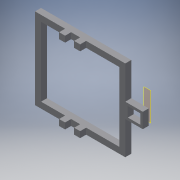
# Autodesk Inventor part: back_pack_side_3
Saved by Autodesk Inventor 2016 (Build 200138000, 138)
## iProperties
Created: 2016-06-09
Part Number: back_pack_side_3
Material: Generic
Document SubType Name: Modeling
Designer: ajar021
Density: 1 g/cm^3
Appearance: Default
Author: ajar021
Autodesk Inventor part; units mm, degrees
ref_plane "YZ Plane" through (0, 0, 0) normal (1, 0, 0) x (0, 1, 0)
ref_plane "XZ Plane" through (0, 0, 0) normal (0, 1, 0) x (-1, 0, 0)
ref_plane "XY Plane" through (0, 0, 0) normal (0, 0, 1) x (1, 0, 0)
ref_plane "Work Plane1" through (0, -1.5, -1) normal (0, 0, 1) x (1, 0, 0)
sketch "Sketch1" plane through (0, -1.5, -1) normal (0, 0, 1) x (1, 0, 0)
  line L0 (-2.8412, 5.5) -> (-2.8412, 7.5) projected
  line L1 (-2.8412, 5.5) -> (-2.8412, 7.5) projected
  line L2 (-2.8412, 5.5) -> (-2.8412, 7.5) projected
  line L3 (-2.8412, 7.5) -> (0, 7.5) projected
  line L4 (-2.8412, 5.5) -> (0, 5.5)
  line L5 (0, 5.5) -> (0, 7.5)
  line L6 (0, 7.5) -> (-2.8412, 7.5)
  line L7 (-2.8412, 7.5) -> (-2.8412, 5.5)
  line L8 (-2.8412, 7.5) -> (-2.8412, 9)
  line L9 (-2.8412, 9) -> (-4.3412, 9)
  line L10 (0, 5.5) -> (0, 4)
  line L11 (0, 4) -> (1.5, 4)
  line L12 (1.5, 4) -> (-4.3412, 4)
  line L13 (-4.3412, 4) -> (-4.3412, 9)
  line L14 (-4.3412, 9) -> (1.5, 9)
  line L15 (1.5, 9) -> (1.5, 4)
  line L16 (-4.3412, 4) -> (-4.3412, -7)
  line L17 (-4.3412, -7) -> (-34.3412, -7)
  line L18 (-4.3412, 9) -> (-4.3412, 20)
  line L19 (-4.3412, 20) -> (-34.3412, 20)
  line L20 (-34.3412, 20) -> (-34.3412, -7)
  line L21 (-4.3412, -7) -> (-4.3412, -5)
  line L22 (-4.3412, -5) -> (-6.3412, -5)
  line L23 (-34.3412, 20) -> (-34.3412, 18)
  line L24 (-34.3412, 18) -> (-32.3412, 18)
  line L25 (-6.3412, -5) -> (-32.3412, -5)
  line L26 (-32.3412, -5) -> (-32.3412, 18)
  line L27 (-32.3412, 18) -> (-6.3412, 18)
  line L28 (-6.3412, 18) -> (-6.3412, -5)
  point P0 (0, 1.5)
  point P1 (-0.8412, 6.5)
  dimension "d0" = 1.5
  dimension "d1" = 1.5
  dimension "d2" = 1.5
  dimension "d3" = 1.5
  dimension "d4" = 11
  dimension "d5" = 30
  dimension "d6" = 11
  dimension "d7" = 2
  dimension "d8" = 2
  dimension "d9" = 2
  dimension "d10" = 2
  constraints: 50 end point, 11 perpendicular, 6 parallel, 3 horizontal, 3 vertical, 2 point on line
  measures "d0" distance of L6.end L8.end
  measures "d1" distance of L8.end L9.end
  measures "d2" distance of L4.end L10.end
  measures "d3" distance of L10.end L11.end
  measures "d4" distance of L12.end L16.end
  measures "d5" distance of L16.end L17.end
  measures "d6" distance of L9.end L18.end
  measures "d7" distance of L16.end L21.end
  measures "d8" distance of L21.end L22.end
  measures "d9" distance of L19.end L23.end
  measures "d10" distance of L23.end L24.end
extrude "Extrusion1" add sketch "Sketch1" along normal blind 2 contours L4 L10 L12 L13 L9 L8 L0 | L8 L14 L15 L11 L10 L5 L3 | L13 L16 L22 L28 L27 L24 L20 L19 L18 | L16 L17 L20 L24 L26 L25 L22
sketch "Sketch2" plane through (0, -1.5, 1) normal (0, 0, 1) x (1, 0, 0)
  line L0 (-34.3412, -7) -> (-4.3412, -7) projected
  line L1 (-4.3412, 20) -> (-34.3412, 20) projected
  line L2 (-6.3412, -5) -> (-19.3412, -5)
  line L3 (-6.3412, -5) -> (-32.3412, -5) projected
  line L4 (-19.3412, -5) -> (-22.3412, -5)
  line L5 (-6.3412, 18) -> (-19.3412, 18)
  line L6 (-32.3412, 18) -> (-6.3412, 18) projected
  line L7 (-19.3412, 18) -> (-22.3412, 18)
  line L8 (-22.3412, -5) -> (-24.3412, -5)
  line L9 (-24.3412, -5) -> (-24.3412, -7)
  line L10 (-24.3412, -7) -> (-22.3412, -7)
  line L11 (-22.3412, -7) -> (-22.3412, -5)
  line L12 (-22.3412, 18) -> (-24.3412, 18)
  line L13 (-24.3412, 18) -> (-24.3412, 20)
  line L14 (-24.3412, 20) -> (-22.3412, 20)
  line L15 (-22.3412, 20) -> (-22.3412, 18)
  line L16 (-19.3412, 18) -> (-17.3412, 18)
  line L17 (-17.3412, 18) -> (-17.3412, 20)
  line L18 (-17.3412, 20) -> (-19.3412, 20)
  line L19 (-19.3412, 20) -> (-19.3412, 18)
  line L20 (-19.3412, -5) -> (-17.3412, -5)
  line L21 (-17.3412, -5) -> (-17.3412, -7)
  line L22 (-17.3412, -7) -> (-19.3412, -7)
  line L23 (-19.3412, -7) -> (-19.3412, -5)
  point P0 (0, 1.5)
  dimension "d13" = 13
  dimension "d14" = 3
  dimension "d15" = 2
  dimension "d16" = 2
  dimension "d17" = 2
  dimension "d18" = 2
  constraints: 40 end point, 8 parallel, 6 point on line, 4 horizontal, 4 perpendicular, 2 midpoint
  measures "d13" distance of L2.start L2.end
  measures "d14" distance of L2.end L4.end
  measures "d15" distance of L10.end L9.end
  measures "d16" distance of L13.end L14.end
  measures "d17" distance of L18.end L17.end
  measures "d18" distance of L21.end L22.end
extrude "Extrusion2" add sketch "Sketch2" along normal blind 2 contours L9 L3 L11 L0 | L23 L2 L21 L0 | L17 L5 L19 L1 | L15 L6 L13 L1
sketch "Sketch3" plane through (0, -1.5, 1) normal (0, 0, 1) x (1, 0, 0)
  line L0 (-2.8412, 5.5) -> (-2.8412, 7.5) projected
  line L1 (-2.8412, 7.5) -> (0, 7.5) projected
  line L2 (0, 7.5) -> (0, 5.5) projected
  line L3 (0, 5.5) -> (-2.8412, 5.5) projected
  line L4 (-2.8412, 7.5) -> (-2.8412, 8.15)
  line L5 (-2.8412, 8.15) -> (-3.4912, 8.15)
  line L6 (-2.8412, 5.5) -> (0, 5.5) projected
  line L7 (0, 5.5) -> (0, 4.85)
  line L8 (0, 4.85) -> (0.65, 4.85)
  line L9 (0.65, 4.85) -> (-3.4912, 4.85)
  line L10 (-3.4912, 4.85) -> (-3.4912, 8.15)
  line L11 (-3.4912, 8.15) -> (0.65, 8.15)
  line L12 (0.65, 8.15) -> (0.65, 4.85)
  point P0 (0, 1.5)
  dimension "d21" = 0.65
  dimension "d22" = 0.65
  dimension "d23" = 0.65
  dimension "d24" = 0.65
  constraints: 16 end point, 2 horizontal, 2 parallel, 2 perpendicular, 2 vertical
  measures "d21" distance of L0.end L4.end
  measures "d22" distance of L4.end L5.end
  measures "d23" distance of L2.end L7.end
  measures "d24" distance of L7.end L8.end
extrude "Extrusion3" cut sketch "Sketch3" against normal up to next contours L3 L7 L9 L10 L5 L4 L0 | L4 L11 L12 L8 L7 L2 L1
equation "\"d6\" = d4"
equation "\"d21\" = d24"
equation "\"d22\" = d24"
equation "\"d23\" = d24"
body "Solid1"
